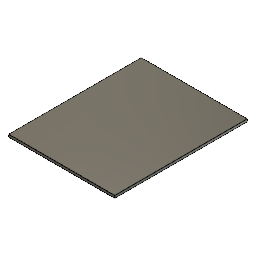
Front_ground v3 (Autodesk Fusion 360 design; units mm, degrees)
Autodesk Fusion 360 part; units mm, degrees
box "BoxPrimitive1" add length 100 width 80 height 2 placed x (0, 0, -1) y (-1, 0, 0) z (0, 1, 0) at (30, 0, 25)
